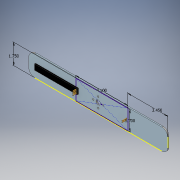
# Autodesk Inventor part: Base
Saved by Autodesk Inventor 2016 (Build 200138000, 138)
## iProperties
Created: 2017-12-06
Part Number: Base
Material: Generic
Document SubType Name: Modeling
Designer: student
Density: 1 g/cm^3
Appearance: Default
Author: student
Autodesk Inventor part; units mm, degrees
ref_plane "YZ Plane" through (0, 0, 0) normal (1, 0, 0) x (0, 1, 0)
ref_plane "XZ Plane" through (0, 0, 0) normal (0, 1, 0) x (-1, 0, 0)
ref_plane "XY Plane" through (0, 0, 0) normal (0, 0, 1) x (1, 0, 0)
sketch "Sketch1" plane through (0, 0, 0) normal (0, 0, 1) x (1, 0, 0)
  line L0 (0, 0) -> (304.8, 0)
  line L1 (304.8, 0) -> (304.8, 45.72)
  line L2 (304.8, 45.72) -> (0, 45.72)
  line L3 (0, 45.72) -> (0, 0)
  dimension "d0" = 304.8
  dimension "d1" = 45.72
  constraints: 8 end point, 2 parallel, 1 horizontal, 1 perpendicular
  measures "d0" distance of L2.end L1.end
  measures "d1" distance of L1.end L0.end
extrude "Extrusion1" add sketch "Sketch1" along normal blind 2.794
sketch "Sketch2" plane through (0, 0, 2.794) normal (0, 0, 1) x (1, 0, 0)
  line L0 (114.3, 0) -> (190.5, 0)
  line L1 (190.5, 0) -> (190.5, 35.56)
  line L2 (190.5, 35.56) -> (114.3, 35.56)
  line L3 (114.3, 35.56) -> (114.3, 0)
  line L4 (114.3, 0) -> (190.5, 35.56) construction
  line L5 (190.5, 0) -> (114.3, 35.56) construction
  line L6 (108.6972, 16.51) -> (14.7172, 16.51)
  line L7 (14.7172, 16.51) -> (14.7172, 28.5496)
  line L8 (14.7172, 28.5496) -> (108.6972, 28.5496)
  line L9 (108.6972, 28.5496) -> (108.6972, 16.51)
  line L10 (108.6972, 16.51) -> (14.7172, 28.5496) construction
  line L11 (14.7172, 16.51) -> (108.6972, 28.5496) construction
  circle A0 centre (106.812, 26.4905) radius 0.7825
  line L12 (14.7172, 13.843) -> (108.6972, 25.8826) construction
  circle A1 centre (106.812, 23.8235) radius 0.7825
  line L13 (14.7172, 11.176) -> (108.6972, 23.2156) construction
  circle A2 centre (106.812, 21.1565) radius 0.7825
  line L14 (14.7172, 8.509) -> (108.6972, 20.5486) construction
  circle A3 centre (106.812, 18.4895) radius 0.7825
  line L15 (0, 0) -> (304.8, 0) projected
  line L16 (0, 45.72) -> (0, 0) projected
  point P0 (152.4, 17.78)
  point P1 (61.7072, 22.5298)
  dimension "d4" = 76.2
  dimension "d5" = 35.56
  dimension "d6" = 93.98
  dimension "d7" = 12.0396
  dimension "d10" = 2.667
  dimension "d56" = 16.51
  dimension "d57" = 14.7172
  dimension "d58" = 2.0591
  dimension "d59" = 1.8853
  dimension "d60" = 1.102
  constraints: 30 end point, 4 centre point, 4 midpoint, 4 parallel, 2 horizontal, 2 perpendicular, 1 vertical, 15 other
  measures "d4" distance of L2.end L1.end
  measures "d5" distance of L1.end L0.end
  measures "d6" distance of L7.end L8.end
  measures "d7" distance of L6.end L7.end
  measures "d10" distance of L6.end L12.start
  measures "d56" distance between parallel lines of L15 L6
  measures "d57" distance between parallel lines of L16 L7
  measures "d58" distance from line of L8 A0.centre
  measures "d59" distance from line of L9 A1.centre
extrude "Extrusion2" add sketch "Sketch2" along normal blind 10.16 contours A0 | A1 | A2 | A3
sketch "Sketch3" plane through (0, 0, 2.794) normal (0, 0, 1) x (1, 0, 0)
  line L0 (114.3, 0) -> (190.5, 0)
  line L1 (190.5, 0) -> (190.5, 35.56)
  line L2 (190.5, 35.56) -> (114.3, 35.56)
  line L3 (114.3, 35.56) -> (114.3, 0)
  line L4 (114.3, 0) -> (190.5, 35.56) construction
  line L5 (190.5, 0) -> (114.3, 35.56) construction
  line L6 (108.6972, 16.4402) -> (14.7172, 16.4401)
  line L7 (14.7172, 16.4401) -> (14.7172, 28.4797)
  line L8 (14.7172, 28.4797) -> (108.6972, 28.4798)
  line L9 (108.6972, 28.4798) -> (108.6972, 16.4402)
  line L10 (108.6972, 16.4402) -> (14.7172, 28.4797) construction
  line L11 (14.7172, 16.4401) -> (108.6972, 28.4798) construction
  circle A0 centre (106.812, 26.4207) radius 0.7825
  line L12 (14.7172, 13.7731) -> (108.6972, 25.8128) construction
  circle A1 centre (106.812, 23.7537) radius 0.7825
  line L13 (14.7172, 11.1061) -> (108.6972, 23.1458) construction
  circle A2 centre (106.812, 21.0867) radius 0.7825
  line L14 (14.7172, 8.4391) -> (108.6972, 20.4788) construction
  circle A3 centre (106.812, 18.4197) radius 0.7825
  line L15 (304.8, 45.72) -> (0, 45.72) projected
  line L16 (0, 45.72) -> (0, 0) projected
  line L17 (0, 0) -> (304.8, 0) projected
  point P0 (152.4, 17.78)
  dimension "d17" = 76.2
  dimension "d18" = 35.56
  dimension "d19" = 93.98
  dimension "d20" = 12.0396
  dimension "d21" = 2.667
  dimension "d63" = 2.0591
  dimension "d64" = 1.8853
  dimension "d68" = 16.4401
  constraints: 30 end point, 4 centre point, 4 parallel, 2 horizontal, 2 midpoint, 2 perpendicular, 1 vertical, 15 other
  measures "d17" distance of L2.end L1.end
  measures "d18" distance of L1.end L0.end
  measures "d19" distance of L7.end L8.end
  measures "d20" distance of L6.end L7.end
  measures "d21" distance of L6.end L12.start
  measures "d63" distance from line of L8 A0.centre
  measures "d64" distance from line of L9 A0.centre
  measures "d68" distance between parallel lines of L17 L6
extrude "Extrusion3" add sketch "Sketch3" along normal blind 2.54 contours L6 L7 L8 L9
sketch "Sketch5" plane through (0, 0, 2.794) normal (0, 0, 1) x (1, 0, 0)
  circle A0 centre (106.812, 23.8235) radius 0.7825 projected
  circle A1 centre (106.812, 21.1565) radius 0.7825 projected
  circle A2 centre (214.4081, 23.402) radius 0.7825
  circle A3 centre (214.4081, 20.735) radius 0.7825
  line L0 (108.6972, 16.4402) -> (108.6972, 28.4798) projected
  point P0 (0, 0)
  dimension "d65" = 107.5969
  dimension "d66" = 105.7108
  dimension "d67" = 107.5961
  constraints: 2 centre point
  measures "d65" distance between centres of A0 A2
  measures "d66" distance from line of L0 A2.centre
  measures "d67" horizontal distance of A0.centre A3.centre
extrude "Extrusion4" add sketch "Sketch5" along normal mid plane 19.05 contours A2 | A3
sketch "Sketch6" plane through (0, 0, 2.794) normal (0, 0, 1) x (1, 0, 0)
  circle A0 centre (152.4, 33.7185) radius 1.6891
  circle A1 centre (152.4, 12.0015) radius 1.6891
  circle A2 centre (163.2585, 22.86) radius 1.6891
  circle A3 centre (141.5415, 22.86) radius 1.6891
  circle A4 centre (152.4, 22.86) radius 4.699
  line L0 (304.8, 45.72) -> (0, 45.72) projected
  line L1 (0, 45.72) -> (0, 0) projected
  dimension "d37" = 3.3782
  dimension "d38" = 3.3782
  dimension "d39" = 3.3782
  dimension "d40" = 3.3782
  dimension "d47" = 9.398
  constraints: 5 centre point
  measures "d37" diameter of A0
  measures "d38" diameter of A1
  measures "d39" diameter of A2
  measures "d40" diameter of A3
  measures "d47" diameter of A4
extrude "Extrusion5" cut sketch "Sketch6" against normal blind 8.89
fillet "Fillet1" radius 12.7 4 edges at (304.8, 0, 1.397) (304.8, 45.72, 1.397) (0, 0, 1.397) (0, 45.72, 1.397)
sketch "Sketch8" plane through (0, 0, 0) normal (0, 0, -1) x (-1, 0, 0)
  line L0 (-177.9476, 6.2522) -> (-187.8536, 6.2522)
  line L1 (-187.8536, 6.2522) -> (-187.8536, 30.3822)
  line L2 (-187.8536, 30.3822) -> (-177.9476, 30.3822)
  line L3 (-177.9476, 30.3822) -> (-177.9476, 6.2522)
  point P0 (0, 0)
  dimension "d48" = 9.906
  dimension "d49" = 24.13
  constraints: 8 end point, 2 parallel, 1 horizontal, 1 perpendicular
  measures "d48" distance of L1.end L2.end
  measures "d49" distance of L0.end L1.end
extrude "Extrusion6" add sketch "Sketch8" along normal blind 3.2258
sketch "Sketch9" plane through (0, 0, 2.794) normal (0, 0, 1) x (1, 0, 0)
  line L0 (102.87, 1.27) -> (217.17, 1.27)
  line L1 (217.17, 1.27) -> (217.17, 44.45)
  line L2 (217.17, 44.45) -> (102.87, 44.45)
  line L3 (102.87, 44.45) -> (102.87, 1.27)
  line L4 (102.87, 1.27) -> (217.17, 44.45) construction
  line L5 (217.17, 1.27) -> (102.87, 44.45) construction
  line L6 (12.7, 0) -> (292.1, 0) projected
  line L7 (304.8, 12.7) -> (304.8, 33.02) projected
  point P0 (160.02, 22.86)
  dimension "d69" = 114.3
  dimension "d70" = 43.18
  dimension "d76" = 44.45
  dimension "d77" = 87.63
  constraints: 12 end point, 2 midpoint, 2 parallel, 1 horizontal, 1 perpendicular
  measures "d69" distance of L2.end L1.end
  measures "d70" distance of L1.end L0.end
  measures "d76" distance between parallel lines of L6 L2
  measures "d77" distance between parallel lines of L7 L1
body "Solid1"
